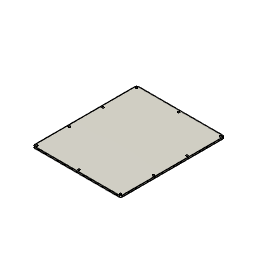
Lid - Standard (Autodesk Fusion 360 design; units mm, degrees)
Autodesk Fusion 360 part; units mm, degrees
note: some values were not read from the file. Set by a fixed rule: which sketch regions a step uses.
sketch "Sketch1" plane through (0, 0, 123.8) normal (0, 0, 1) x (-1, 0, 0)
  line L0 (8.2, -139) -> (-71.5, -139)
  arc A0 (-81.5, -129) -> (-71.5, -139) centre (-71.5, -129) ccw
  line L1 (-81.5, -129) -> (-81.5, 46.7937)
  arc A1 (-71.5, 56.7937) -> (-81.5, 46.7937) centre (-71.5, 46.7937) ccw
  line L2 (-71.5, 56.7937) -> (71.5, 56.7937)
  arc A2 (81.5, 46.7937) -> (71.5, 56.7937) centre (71.5, 46.7937) ccw
  line L3 (81.5, 46.7937) -> (81.5, -129)
  arc A3 (71.5, -139) -> (81.5, -129) centre (71.5, -129) ccw
  line L4 (71.5, -139) -> (68.8, -139)
  line L5 (68.8, -147) -> (86.5, -147)
  arc A4 (86.5, -147) -> (89.5, -144) centre (86.5, -144) ccw
  line L6 (89.5, -144) -> (89.5, 61.7937)
  arc A5 (89.5, 61.7937) -> (86.5, 64.7937) centre (86.5, 61.7937) ccw
  line L7 (86.5, 64.7937) -> (-86.5, 64.7937)
  arc A6 (-86.5, 64.7937) -> (-89.5, 61.7937) centre (-86.5, 61.7937) ccw
  line L8 (-89.5, 61.7937) -> (-89.5, -144)
  arc A7 (-89.5, -144) -> (-86.5, -147) centre (-86.5, -144) ccw
  circle A8 centre (0, -143) radius 1.9
  circle A9 centre (85.5, -74.3226) radius 1.9
  circle A10 centre (85.5, 60.7937) radius 1.9
  circle A11 centre (-85.5, -5.6453) radius 1.9
  circle A12 centre (85.5, -143) radius 1.9
  circle A13 centre (0, 60.7937) radius 1.9
  circle A14 centre (-85.5, -74.3226) radius 1.9
  circle A15 centre (-85.5, 60.7937) radius 1.9
  circle A16 centre (85.5, -5.6453) radius 1.9
  circle A17 centre (-85.5, -143) radius 1.9
  line L9 (68.8, -147) -> (66.6132, -147)
  line L10 (66.6132, -147) -> (8.2, -147)
  line L11 (68.8, -139) -> (68.8, -147)
  line L12 (-86.5, -147) -> (8.2, -147)
  line L13 (8.2, -147) -> (8.2, -139)
  constraint coincident L5.start L9.start
extrude "Extrude1" add sketch "Sketch1" along normal blind 3
sketch "Sketch2" plane through (0, 0, 126.8) normal (0, 0, 1) x (-1, 0, 0)
  circle A0 centre (0, -143) radius 1.9
  circle A1 centre (0, 60.7937) radius 1.9
  circle A2 centre (85.5, -143) radius 1.9
  circle A3 centre (-85.5, 60.7937) radius 1.9
  circle A4 centre (-85.5, -74.3226) radius 1.9
  circle A5 centre (85.5, 60.7937) radius 1.9
  circle A6 centre (85.5, -74.3226) radius 1.9
  circle A7 centre (-85.5, -143) radius 1.9
  circle A8 centre (-85.5, -5.6453) radius 1.9
  circle A9 centre (85.5, -5.6453) radius 1.9
  line L0 (-86.5, -147) -> (86.5, -147)
  arc A10 (86.5, -147) -> (89.5, -144) centre (86.5, -144) ccw
  line L1 (89.5, -144) -> (89.5, 61.7937)
  arc A11 (89.5, 61.7937) -> (86.5, 64.7937) centre (86.5, 61.7937) ccw
  line L2 (86.5, 64.7937) -> (-86.5, 64.7937)
  arc A12 (-86.5, 64.7937) -> (-89.5, 61.7937) centre (-86.5, 61.7937) ccw
  line L3 (-89.5, 61.7937) -> (-89.5, -144)
  arc A13 (-89.5, -144) -> (-86.5, -147) centre (-86.5, -144) ccw
  line L4 (89.4, -144) -> (89.4, 61.7937)
  arc A14 (89.4, 61.7937) -> (86.5, 64.6937) centre (86.5, 61.7937) ccw
  line L5 (86.5, 64.6937) -> (-86.5, 64.6937)
  arc A15 (-86.5, 64.6937) -> (-89.4, 61.7937) centre (-86.5, 61.7937) ccw
  line L6 (-89.4, 61.7937) -> (-89.4, -144)
  arc A16 (-89.4, -144) -> (-86.5, -146.9) centre (-86.5, -144) ccw
  line L7 (-86.5, -146.9) -> (86.5, -146.9)
  arc A17 (86.5, -146.9) -> (89.4, -144) centre (86.5, -144) ccw
  dimension "d970" = -0.1
extrude "Extrude2" cut sketch "Sketch2" against normal blind 4 contours L0 A10 L1 A11 L2 A12 L3 A13
